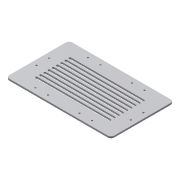
# Autodesk Inventor part: BottomFrontPanel
Saved by Autodesk Inventor 2014 (Build 180170000, 170)
## iProperties
Created: 2014-08-11
Part Number: BottomFrontPanel
Material: Generic
Document SubType Name: Modeling
Designer: Peele
Density: 1 g/cm^3
Appearance: White
Author: Peele
Autodesk Inventor part; units mm, degrees
ref_plane "YZ Plane" through (0, 0, 0) normal (1, 0, 0) x (0, 1, 0)
ref_plane "XZ Plane" through (0, 0, 0) normal (0, 1, 0) x (-1, 0, 0)
ref_plane "XY Plane" through (0, 0, 0) normal (0, 0, 1) x (1, 0, 0)
sketch "Sketch1" plane through (0, 0, 0) normal (0, 0, 1) x (1, 0, 0)
  line L0 (-100, -50) -> (100, -50)
  line L1 (100, -50) -> (100, 50)
  line L2 (100, 50) -> (-100, 50)
  line L3 (-100, 50) -> (-100, -50)
  line L4 (-100, -50) -> (100, 50) construction
  line L5 (100, -50) -> (-100, 50) construction
  point P0 (0, 0)
  dimension "d0" = 200
  dimension "d1" = 100
  constraints: 12 end point, 2 midpoint, 2 parallel, 1 horizontal, 1 perpendicular
  measures "d0" distance of L1.end L2.end
  measures "d1" distance of L0.end L1.end
extrude "Extrusion1" add sketch "Sketch1" along normal blind 4
sketch "Sketch2" plane through (0, 0, 4) normal (0, 0, 1) x (1, 0, 0)
  line L0 (-100, -50) -> (-125, -25)
  line L1 (-125, -25) -> (-125, 25)
  line L2 (-125, 25) -> (-100, 50)
  line L3 (-100, 50) -> (-75, 75)
  line L4 (-75, 75) -> (-30, 75)
  line L5 (-30, 75) -> (-5, 50)
  line L6 (-100, -50) -> (-75, -75)
  line L7 (-75, -75) -> (-30, -75)
  line L8 (-30, -75) -> (-5, -50)
  line L9 (-5, 50) -> (-5, -50)
  line L10 (100, 50) -> (75, 75)
  line L11 (75, 75) -> (30, 75)
  line L12 (30, 75) -> (5, 50)
  line L13 (100, 50) -> (5, 50)
  line L14 (100, -50) -> (5, -50)
  line L15 (5, -50) -> (30, -75)
  line L16 (30, -75) -> (75, -75)
  line L17 (75, -75) -> (100, -50)
  circle A0 centre (-67.5, 62.5) radius 2
  circle A1 centre (-37.5, 62.5) radius 2
  circle A2 centre (37.5, 62.5) radius 2
  circle A3 centre (67.5, 62.5) radius 2
  circle A4 centre (37.5, -62.5) radius 2
  circle A5 centre (67.5, -62.5) radius 2
  circle A6 centre (-67.5, -62.5) radius 2
  circle A7 centre (-37.5, -62.5) radius 2
  circle A8 centre (-112.5, -15) radius 2
  circle A9 centre (-112.5, 15) radius 2
  line L18 (-100, -50) -> (100, -50) projected
  line L19 (100, -50) -> (100, 50) projected
  line L20 (100, -50) -> (100, 50)
  line L21 (125, 25) -> (125, -25)
  line L22 (125, -25) -> (100, -50)
  line L23 (125, 25) -> (100, 50)
  circle A10 centre (112.5, 15) radius 2
  circle A11 centre (112.5, -15) radius 2
  point P0 (0, 0)
  dimension "d6" = 45
  dimension "d8" = 30
  dimension "d9" = 30
  dimension "d11" = 30
  dimension "d13" = 25
  dimension "d14" = 7.5
  dimension "d15" = 7.5
  dimension "d16" = 50
  dimension "d17" = 10
  dimension "d18" = 12.5
  dimension "d19" = 4
  dimension "d20" = 12.5
  dimension "d21" = 12.5
  dimension "d24" = 12.5
  constraints: 44 end point, 14 equal length, 12 centre point, 11 equal radius, 8 horizontal alignment, 6 vertical alignment, 5 perpendicular, 4 collinear, 3 parallel, 2 horizontal, 1 point on line
  measures "d6" distance of L3.end L4.end
  measures "d8" distance of A3.centre A2.centre
  measures "d9" distance of A0.centre A1.centre
  measures "d11" distance of A9.centre A8.centre
  measures "d13" distance between parallel lines of L11 L13
  measures "d14" horizontal distance of L11.end A2.centre
  measures "d15" horizontal distance of L4.end A1.centre
  measures "d16" distance of L0.end L1.end
  measures "d17" vertical distance of L1.end A9.centre
  measures "d18" distance from line of L1 A9.centre
  measures "d19" diameter of A3
  measures "d20" distance from line of A3.centre L13
  measures "d21" distance from line of A5.centre L14
  measures "d24" distance from line of L19 A11.centre
extrude "Extrusion2" add sketch "Sketch2" against normal blind 4
sketch "Sketch3" plane through (0, 0, 4) normal (0, 0, 1) x (1, 0, 0)
  line L0 (-5, -50) -> (5, -50) projected
  line L1 (5, -50) -> (30, -75) projected
  line L2 (75, -75) -> (125, -25) projected
  line L3 (125, 25) -> (75, 75) projected
  line L4 (30, 75) -> (5, 50) projected
  line L5 (5, 50) -> (-5, 50) projected
  line L6 (-5, 50) -> (-30, 75) projected
  line L7 (-75, 75) -> (-125, 25) projected
  line L8 (-125, -25) -> (-75, -75) projected
  line L9 (-30, -75) -> (-5, -50) projected
  line L10 (-75, 75) -> (-125, 75)
  line L11 (-125, 75) -> (-125, 25)
  line L12 (-125, 25) -> (-75, 25)
  line L13 (-75, 25) -> (-75, 75)
  line L14 (-125, -25) -> (-75, -25)
  line L15 (-75, -25) -> (-75, -75)
  line L16 (-75, -75) -> (-125, -75)
  line L17 (-125, -75) -> (-125, -25)
  line L18 (75, -75) -> (125, -75)
  line L19 (125, -75) -> (125, -25)
  line L20 (125, -25) -> (75, -25)
  line L21 (75, -25) -> (75, -75)
  line L22 (75, 75) -> (125, 75)
  line L23 (125, 75) -> (125, 25)
  line L24 (125, 25) -> (75, 25)
  line L25 (75, 25) -> (75, 75)
  line L26 (30, 75) -> (-30, 75)
  line L27 (-30, 75) -> (-30, 50)
  line L28 (-30, 50) -> (30, 50)
  line L29 (30, 50) -> (30, 75)
  line L30 (30, -75) -> (-30, -75)
  line L31 (-30, -75) -> (-30, -50)
  line L32 (-30, -50) -> (30, -50)
  line L33 (30, -50) -> (30, -75)
  point P0 (0, 0)
  constraints: 48 end point, 12 parallel, 6 horizontal, 6 perpendicular, 2 collinear
extrude "Extrusion3" add sketch "Sketch3" against normal blind 4 contours L0 L1 L30 L9 | L2 L19 L18 | L3 L22 L23 | L4 L5 L6 L26 | L7 L11 L10 | L8 L16 L17
fillet "Fillet1" radius 8 4 edges at (-125, -75, 2) (125, -75, 2) (125, 75, 2) (-125, 75, 2)
sketch "Sketch4" plane through (0, 0, 4) normal (0, 0, 1) x (1, 0, 0)
  line L0 (-125, 67) -> (-125, -67) projected
  line L1 (-117, -75) -> (117, -75) projected
  line L2 (-87.5, 40) -> (87.5, 40) construction
  line L3 (-87.5, 37.5) -> (87.5, 37.5)
  line L4 (87.5, 42.5) -> (-87.5, 42.5)
  arc A0 (-87.5, 42.5) -> (-87.5, 37.5) centre (-87.5, 40) ccw
  arc A1 (87.5, 37.5) -> (87.5, 42.5) centre (87.5, 40) ccw
  line L5 (-87.5, 27.5) -> (87.5, 27.5)
  line L6 (87.5, 32.5) -> (-87.5, 32.5)
  arc A2 (-87.5, 32.5) -> (-87.5, 27.5) centre (-87.5, 30) ccw
  arc A3 (87.5, 27.5) -> (87.5, 32.5) centre (87.5, 30) ccw
  line L7 (-87.5, 17.5) -> (87.5, 17.5)
  line L8 (87.5, 22.5) -> (-87.5, 22.5)
  arc A4 (-87.5, 22.5) -> (-87.5, 17.5) centre (-87.5, 20) ccw
  arc A5 (87.5, 17.5) -> (87.5, 22.5) centre (87.5, 20) ccw
  line L9 (-87.5, 7.5) -> (87.5, 7.5)
  line L10 (87.5, 12.5) -> (-87.5, 12.5)
  arc A6 (-87.5, 12.5) -> (-87.5, 7.5) centre (-87.5, 10) ccw
  arc A7 (87.5, 7.5) -> (87.5, 12.5) centre (87.5, 10) ccw
  line L11 (-87.5, -2.5) -> (87.5, -2.5)
  line L12 (87.5, 2.5) -> (-87.5, 2.5)
  arc A8 (-87.5, 2.5) -> (-87.5, -2.5) centre (-87.5, 0) ccw
  arc A9 (87.5, -2.5) -> (87.5, 2.5) centre (87.5, 0) ccw
  line L13 (-87.5, -12.5) -> (87.5, -12.5)
  line L14 (87.5, -7.5) -> (-87.5, -7.5)
  arc A10 (-87.5, -7.5) -> (-87.5, -12.5) centre (-87.5, -10) ccw
  arc A11 (87.5, -12.5) -> (87.5, -7.5) centre (87.5, -10) ccw
  line L15 (-87.5, -22.5) -> (87.5, -22.5)
  line L16 (87.5, -17.5) -> (-87.5, -17.5)
  arc A12 (-87.5, -17.5) -> (-87.5, -22.5) centre (-87.5, -20) ccw
  arc A13 (87.5, -22.5) -> (87.5, -17.5) centre (87.5, -20) ccw
  line L17 (-87.5, -32.5) -> (87.5, -32.5)
  line L18 (87.5, -27.5) -> (-87.5, -27.5)
  arc A14 (-87.5, -27.5) -> (-87.5, -32.5) centre (-87.5, -30) ccw
  arc A15 (87.5, -32.5) -> (87.5, -27.5) centre (87.5, -30) ccw
  line L19 (-87.5, -42.5) -> (87.5, -42.5)
  line L20 (87.5, -37.5) -> (-87.5, -37.5)
  arc A16 (-87.5, -37.5) -> (-87.5, -42.5) centre (-87.5, -40) ccw
  arc A17 (87.5, -42.5) -> (87.5, -37.5) centre (87.5, -40) ccw
  point P0 (0, 0)
  point P1 (0, 40)
  dimension "d30" = 10
  dimension "d35" = 175
  dimension "d36" = 2.5
  dimension "d37" = 87.5
  constraints: 40 end point, 36 point on circle, 18 centre point, 4 tangent, 2 parallel, 1 horizontal alignment, 1 midpoint, 1 vertical, 80 other
  measures "d30" distance of L4.start L6.start
  measures "d35" distance of L2.start L2.end
  measures "d36" radius of A0
  measures "d37" horizontal distance of L2.start point (0, 0)
extrude "Extrusion4" cut sketch "Sketch4" against normal blind 4
equation "\"d9\" = d8"
equation "\"d14\" = -0.5 * d9 + 0.5 * d6"
equation "\"d15\" = d14"
equation "\"d17\" = -0.5 * d11 + 0.5 * d16"
equation "\"d37\" = 0.5 * d35"
body "Solid1"
